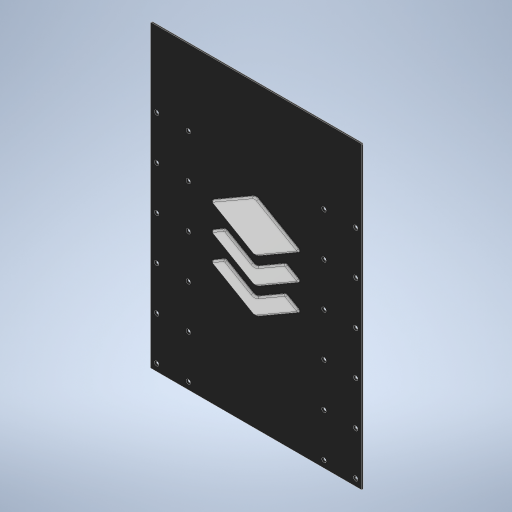
# Autodesk Inventor part: Exterior Side Panels
Saved by Autodesk Inventor 2024 (Build 280153000, 153)
## iProperties
Created: 2024-09-03
Part Number: Exterior Side Panels
Material: PET Plastic
Document SubType Name: Modeling
Designer: Ishaan
Density: 1.541 g/cm^3
Appearance: Polycarbonate - Clear
Author: Ishaan
Autodesk Inventor part; units mm, degrees
ref_plane "YZ Plane" through (0, 0, 0) normal (1, 0, 0) x (0, 1, 0)
ref_plane "XZ Plane" through (0, 0, 0) normal (0, 1, 0) x (-1, 0, 0)
ref_plane "XY Plane" through (0, 0, 0) normal (0, 0, 1) x (1, 0, 0)
sketch "Sketch1" plane through (0, 0, 0) normal (0, 0, 1) x (1, 0, 0)
  line L0 (234.35, -332.175) -> (-234.35, -332.175) construction
  line L1 (-234.35, -332.175) -> (-234.35, 332.175) construction
  line L2 (-234.35, 332.175) -> (234.35, 332.175) construction
  line L3 (234.35, 332.175) -> (234.35, -332.175) construction
  line L4 (234.35, -332.175) -> (-234.35, 332.175) construction
  line L5 (-234.35, -332.175) -> (234.35, 332.175) construction
  line L6 (-234.35, 180.525) -> (234.35, 180.525) construction
  line L7 (-220, 164.175) -> (-220, -315.825) construction
  line L8 (0, 332.175) -> (0, -332.175) construction
  line L9 (-150, 164.175) -> (-150, -291.4433) construction
  line L10 (-233.35, 331.175) -> (-233.35, -331.175)
  line L11 (-233.35, -331.175) -> (233.35, -331.175)
  line L12 (233.35, -331.175) -> (233.35, 331.175)
  line L13 (233.35, 331.175) -> (-233.35, 331.175)
  point P0 (0, 0)
  point P1 (-220, 68.175)
  point P2 (220, 164.175)
  point P3 (220, 68.175)
  point P4 (-220, -27.825)
  point P5 (220, -27.825)
  point P6 (-220, -123.825)
  point P7 (220, -123.825)
  point P8 (-220, -219.825)
  point P9 (220, -219.825)
  point P10 (220, -315.825)
  point P11 (-150, 68.175)
  point P12 (-150, -27.825)
  point P13 (-150, -123.825)
  point P14 (-150, -219.825)
  point P15 (-150, -315.825)
  point P16 (150, 164.175)
  point P17 (150, 68.175)
  point P18 (150, -27.825)
  point P19 (150, -123.825)
  point P20 (150, -219.825)
  point P21 (150, -315.825)
  dimension "d0" = 468.7
  dimension "d1" = 664.35
  dimension "d17" = 512.7
  dimension "d25" = 480
  dimension "d26" = 14.35
  dimension "d27" = 16.35
  dimension "d28" = 16.35
  dimension "d31" = 96
  dimension "d34" = 440
  dimension "d37" = 220
  dimension "d38" = 220
  dimension "d39" = 84.35
  dimension "d42" = 96
  dimension "d45" = 300
  dimension "d48" = 84.35
  dimension "d49" = 1
  constraints: 28 end point, 4 horizontal, 4 midpoint, 4 parallel, 4 vertical, 2 coincident, 2 perpendicular, 2 point on line, 1 horizontal alignment, 25 other
  measures "d0" distance of L1.end L2.end
  measures "d1" distance of L0.end L1.end
  measures "d17" distance between parallel lines of L0 L6
  measures "d25" distance of L7.start L7.end
  measures "d26" distance between parallel lines of L7 L1
  measures "d27" distance from line of L6 L7.start
  measures "d28" distance from line of L0 L7.end
  measures "d31" distance of L7.start point (-220, 68.175)
  measures "d34" distance of L7.start point (220, 164.175)
  measures "d37" distance from line of L8 L7.start
  measures "d38" distance from line of point (220, 164.175) L8
  measures "d39" distance between parallel lines of L9 L1
  measures "d42" distance of point (-150, 164.175) point (-150, 68.175)
  measures "d45" distance of point (-150, 164.175) point (150, 164.175)
  measures "d48" distance from line of L3 point (150, 68.175)
  measures "d49" distance between parallel lines of L1 L10
extrude "Extrusion1" add sketch "Sketch1" against normal blind 3
hole "Hole1" at (-220, 164.175, 0) at (-220, -315.825, 0) at (-220, 68.175, 0) at (220, 164.175, 0) at (220, 68.175, 0) at (-220, -27.825, 0) at (220, -27.825, 0) at (-220, -123.825, 0) at (220, -123.825, 0) at (-220, -219.825, 0) at (220, -219.825, 0) at (220, -315.825, 0) at (-150, 164.175, 0) at (-150, 68.175, 0) at (-150, -27.825, 0) at (-150, -123.825, 0) at (-150, -219.825, 0) at (-150, -315.825, 0) at (150, 164.175, 0) at (150, 68.175, 0) at (150, -27.825, 0) at (150, -123.825, 0) at (150, -219.825, 0) at (150, -315.825, 0) direction (0, 0, -1) diameter 5.4 end through all countersink diameter 10 countersink angle 90
sketch "Sketch4" plane through (0, 0, 0) normal (0, 0, 1) x (1, 0, 0)
  line L0 (0, 115.4701) -> (100, 57.735)
  line L1 (100, 57.735) -> (100, -57.735)
  line L2 (100, -57.735) -> (0, -115.4701)
  line L3 (0, -115.4701) -> (-100, -57.735)
  line L4 (-100, -57.735) -> (-100, 57.735)
  line L5 (-100, 57.735) -> (0, 115.4701)
  line L6 (-100, 57.735) -> (0, 0)
  line L7 (0, 0) -> (100, 57.735)
  line L8 (-100, 38.49) -> (0, -19.245)
  line L9 (0, -19.245) -> (100, 38.49)
  line L10 (100, 0) -> (0, -57.735)
  line L11 (0, -57.735) -> (-100, 0)
  line L12 (-100, -19.245) -> (0, -76.98)
  line L13 (0, -76.98) -> (100, -19.245)
  line L14 (-100, 0) -> (-66.6667, 19.245)
  line L15 (100, 0) -> (66.6667, 19.245)
  line L16 (100, -57.735) -> (66.6667, -38.49)
  line L17 (-100, -57.735) -> (-66.6667, -38.49)
  dimension "d57" = 16.6667
  dimension "d58" = 33.3333
  dimension "d59" = 16.6667
  dimension "d60" = 33.3333
  dimension "d61" = 200
  constraints: 37 end point, 10 parallel, 8 point on line, 5 vertical alignment, 2 midpoint, 1 coincident, 1 vertical, 13 other
  measures "d57" distance between parallel lines of L6 L8
  measures "d58" distance between parallel lines of L8 L11
  measures "d59" distance between parallel lines of L11 L12
  measures "d60" distance between parallel lines of L12 L3
  measures "d61" distance between parallel lines of L1 L4
extrude "Extrusion4" cut sketch "Sketch4" against normal blind 1.5 contours L0 L7 L6 L5 | L10 L11 L14 L8 L9 L15 | L2 L3 L17 L12 L13 L16
fillet "Fillet3" radius 12 6 edges at (0, -76.98, -0.75) (0, -57.735, -0.75) (0, 115.4701, -0.75) (0, 0, -0.75) (0, -19.245, -0.75) (0, -115.4701, -0.75)
fillet "Fillet4" radius 6 4 edges at (-66.6667, 19.245, -0.75) (-66.6667, -38.49, -0.75) (66.6667, -38.49, -0.75) (66.6667, 19.245, -0.75)
fillet "Fillet2" radius 4 6 edges at (-100, 57.735, -0.75) (-100, 0, -0.75) (-100, -57.735, -0.75) (100, -57.735, -0.75) (100, 0, -0.75) (100, 57.735, -0.75)
sketch "Sketch5" plane through (0, 0, -1.5) normal (0, 0, 1) x (1, 0, 0)
  arc A0 (94, 54.2709) -> (94, 61.1991) centre (92, 57.735) ccw projected
  line L0 (6, 112.006) -> (94, 61.1991) projected
  arc A1 (6, 112.006) -> (-6, 112.006) centre (0, 101.6136) ccw projected
  line L1 (-94, 61.1991) -> (-6, 112.006) projected
  arc A2 (-94, 61.1991) -> (-94, 54.2709) centre (-92, 57.735) ccw projected
  line L2 (-6, 3.4641) -> (-94, 54.2709) projected
  arc A3 (-6, 3.4641) -> (6, 3.4641) centre (0, 13.8564) ccw projected
  line L3 (94, 54.2709) -> (6, 3.4641) projected
  arc A4 (94, -3.4641) -> (94, 3.4641) centre (92, 0) ccw projected
  line L4 (69.6667, 17.513) -> (94, 3.4641) projected
  arc A5 (69.6667, 17.513) -> (63.6667, 17.513) centre (66.6667, 12.3168) ccw projected
  line L5 (6, -15.7809) -> (63.6667, 17.513) projected
  arc A6 (-6, -15.7809) -> (6, -15.7809) centre (0, -5.3886) ccw projected
  line L6 (-63.6667, 17.513) -> (-6, -15.7809) projected
  arc A7 (-63.6667, 17.513) -> (-69.6667, 17.513) centre (-66.6667, 12.3168) ccw projected
  line L7 (-94, 3.4641) -> (-69.6667, 17.513) projected
  arc A8 (-94, 3.4641) -> (-94, -3.4641) centre (-92, 0) ccw projected
  line L8 (-6, -54.2709) -> (-94, -3.4641) projected
  arc A9 (-6, -54.2709) -> (6, -54.2709) centre (0, -43.8786) ccw projected
  line L9 (94, -3.4641) -> (6, -54.2709) projected
  arc A10 (94, -61.1991) -> (94, -54.2709) centre (92, -57.735) ccw projected
  line L10 (69.6667, -40.2221) -> (94, -54.2709) projected
  arc A11 (69.6667, -40.2221) -> (63.6667, -40.2221) centre (66.6667, -45.4182) ccw projected
  line L11 (6, -73.5159) -> (63.6667, -40.2221) projected
  arc A12 (-6, -73.5159) -> (6, -73.5159) centre (0, -63.1236) ccw projected
  line L12 (-63.6667, -40.2221) -> (-6, -73.5159) projected
  arc A13 (-63.6667, -40.2221) -> (-69.6667, -40.2221) centre (-66.6667, -45.4182) ccw projected
  line L13 (-94, -54.2709) -> (-69.6667, -40.2221) projected
  arc A14 (-94, -54.2709) -> (-94, -61.1991) centre (-92, -57.735) ccw projected
  line L14 (-6, -112.006) -> (-94, -61.1991) projected
  arc A15 (-6, -112.006) -> (6, -112.006) centre (0, -101.6136) ccw projected
  line L15 (94, -61.1991) -> (6, -112.006) projected
  arc A16 (5.875, 111.7894) -> (-5.875, 111.7894) centre (0, 101.6136) ccw
  line L16 (5.875, 111.7894) -> (93.875, 60.9826)
  arc A17 (93.875, 54.4874) -> (93.875, 60.9826) centre (92, 57.735) ccw
  line L17 (93.875, 54.4874) -> (5.875, 3.6806)
  arc A18 (-5.875, 3.6806) -> (5.875, 3.6806) centre (0, 13.8564) ccw
  line L18 (-5.875, 3.6806) -> (-93.875, 54.4874)
  arc A19 (-93.875, 60.9826) -> (-93.875, 54.4874) centre (-92, 57.735) ccw
  line L19 (-93.875, 60.9826) -> (-5.875, 111.7894)
  arc A20 (-63.7917, 17.2965) -> (-69.5417, 17.2965) centre (-66.6667, 12.3168) ccw
  line L20 (-63.7917, 17.2965) -> (-6.125, -15.9974)
  arc A21 (-6.125, -15.9974) -> (6.125, -15.9974) centre (0, -5.3886) ccw
  line L21 (6.125, -15.9974) -> (63.7917, 17.2965)
  arc A22 (69.5417, 17.2965) -> (63.7917, 17.2965) centre (66.6667, 12.3168) ccw
  line L22 (69.5417, 17.2965) -> (93.875, 3.2476)
  arc A23 (93.875, -3.2476) -> (93.875, 3.2476) centre (92, 0) ccw
  line L23 (93.875, -3.2476) -> (5.875, -54.0544)
  arc A24 (-5.875, -54.0544) -> (5.875, -54.0544) centre (0, -43.8786) ccw
  line L24 (-5.875, -54.0544) -> (-93.875, -3.2476)
  arc A25 (-93.875, 3.2476) -> (-93.875, -3.2476) centre (-92, 0) ccw
  line L25 (-93.875, 3.2476) -> (-69.5417, 17.2965)
  arc A26 (-63.7917, -40.4386) -> (-69.5417, -40.4386) centre (-66.6667, -45.4182) ccw
  line L26 (-63.7917, -40.4386) -> (-6.125, -73.7324)
  arc A27 (-6.125, -73.7324) -> (6.125, -73.7324) centre (0, -63.1236) ccw
  line L27 (6.125, -73.7324) -> (63.7917, -40.4386)
  arc A28 (69.5417, -40.4386) -> (63.7917, -40.4386) centre (66.6667, -45.4182) ccw
  line L28 (69.5417, -40.4386) -> (93.875, -54.4874)
  arc A29 (93.875, -60.9826) -> (93.875, -54.4874) centre (92, -57.735) ccw
  line L29 (93.875, -60.9826) -> (5.875, -111.7894)
  arc A30 (-5.875, -111.7894) -> (5.875, -111.7894) centre (0, -101.6136) ccw
  line L30 (-5.875, -111.7894) -> (-93.875, -60.9826)
  arc A31 (-93.875, -54.4874) -> (-93.875, -60.9826) centre (-92, -57.735) ccw
  line L31 (-93.875, -54.4874) -> (-69.5417, -40.4386)
  dimension "d75" = 0.25
  dimension "d76" = 0.25
  dimension "d77" = 0.25
  constraints: 32 end point, 32 point on circle, 16 centre point, 29 other
  measures "d75" distance between parallel lines of L1 L19
  measures "d76" distance between parallel lines of L6 L20
  measures "d77" distance between parallel lines of L12 L26
extrude "Extrusion5" add sketch "Sketch5" along normal blind 5 separate body contours L16 A17 L17 A18 L18 A19 L19 A16 | L20 A21 L21 A22 L22 A23 L23 A24 L24 A25 L25 A20 | L26 A27 L27 A28 L28 A29 L29 A30 L30 A31 L31 A26
chamfer "Chamfer1" distance 3 angle 45 32 edges at (-49.875, -86.386, 3.5) (0, -113.3636, 3.5) (49.875, -86.386, 3.5) (95.75, -57.735, 3.5) (81.7083, -47.463, 3.5) (66.6667, -39.6682, 3.5) (34.9583, -57.0855, 3.5) (0, -75.3736, 3.5) (-34.9583, -57.0855, 3.5) (-66.6667, -39.6682, 3.5) (-81.7083, -47.463, 3.5) (-95.75, -57.735, 3.5) (-49.875, -28.651, 3.5) (0, -55.6286, 3.5) (49.875, -28.651, 3.5) (95.75, 0, 3.5) (81.7083, 10.272, 3.5) (66.6667, 18.0668, 3.5) (34.9583, 0.6495, 3.5) (0, -17.6386, 3.5) (-34.9583, 0.6495, 3.5) (-66.6667, 18.0668, 3.5) (-81.7083, 10.272, 3.5) (-95.75, 0, 3.5) (-49.875, 29.084, 3.5) (0, 2.1064, 3.5) (49.875, 29.084, 3.5) (95.75, 57.735, 3.5) (49.875, 86.386, 3.5) (0, 113.3636, 3.5) (-49.875, 86.386, 3.5) (-95.75, 57.735, 3.5)
fillet "Fillet5" radius 2 2 edges at (-233.35, 331.175, -1.5) (233.35, 331.175, -1.5)
equation "\"d27\" = d28"
equation "\"d38\" = d37"
equation "\"d42\" = d31"
equation "\"d48\" = d39"
equation "\"d58\" = 2 * d57"
equation "\"d59\" = d57"
equation "\"d60\" = d58"
equation "\"d76\" = d75"
equation "\"d77\" = d76"
body "Solid1"
